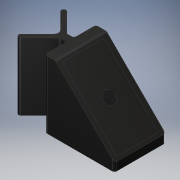
# Autodesk Inventor part: MainHousing
Saved by Autodesk Inventor 2019 (Build 230136000, 136)
## iProperties
Created: 2018-09-02
Part Number: MainHousing
Material: Generic
Document SubType Name: Modeling
Designer: Crater-Windows
Density: 1 g/cm^3
Appearance: Glossy - Black
Author: Crater-Windows
Autodesk Inventor part; units mm, degrees
ref_plane "YZ Plane" through (0, 0, 0) normal (1, 0, 0) x (0, 1, 0)
ref_plane "XZ Plane" through (0, 0, 0) normal (0, 1, 0) x (-1, 0, 0)
ref_plane "XY Plane" through (0, 0, 0) normal (0, 0, 1) x (1, 0, 0)
sketch "Sketch1" plane through (0, 0, 0) normal (1, 0, 0) x (0, 1, 0)
  line L0 (0, 0) -> (150, 0)
  line L1 (150, 0) -> (150, -110)
  line L2 (150, -110) -> (0, -110)
  line L3 (0, -110) -> (0, 0)
  dimension "d0" = 150
  dimension "d1" = 110
  constraints: 8 end point, 2 parallel, 1 horizontal, 1 perpendicular
  measures "d0" distance of L1.end L2.end
  measures "d1" distance of L0.end L1.end
extrude "Extrusion1" add sketch "Sketch1" along normal blind 150
sketch "Sketch2" plane through (0, 0, 0) normal (0, 0, 1) x (1, 0, 0)
  line L0 (0, 0) -> (0, 150) projected
  line L1 (0, 0) -> (150, 0) projected
  line L2 (150, 150) -> (150, 0) projected
  line L3 (0, 150) -> (150, 150) projected
  line L4 (0, 150) -> (150, 150) projected
  line L5 (22.7208, 150) -> (150, 22.7208)
  line L6 (22.7208, 150) -> (202.7208, 150) construction
  line L7 (150, 150) -> (150, 0) projected
  dimension "d4" = 45
  dimension "d6" = 180
  constraints: 4 end point, 2 point on line, 1 equal length, 1 horizontal
  measures "d4" angle of L5 L6
  measures "d6" distance of L5.start L5.end
extrude "Extrusion2" cut sketch "Sketch2" against normal blind 150 contours L3 L2 L5
shell "Shell1" thickness 6 removed faces 1 at (50, 0, -73.3333)
sketch "Sketch3" plane through (22.7208, 150, -110) normal (0.7071068, 0.7071068, 0) x (-0.7071068, 0.7071068, 0)
  line L0 (-7, 100) -> (-173, 100)
  line L1 (-173, 100) -> (-173, 10)
  line L2 (-173, 10) -> (-7, 10)
  line L3 (-7, 10) -> (-7, 100)
  line L4 (0, 110) -> (0, 0) projected
  line L5 (-180, 110) -> (0, 110) projected
  point P0 (-90, 110)
  dimension "d10" = 166
  dimension "d11" = 90
  dimension "d12" = 7
  dimension "d13" = 10
  constraints: 8 end point, 2 parallel, 1 horizontal, 1 perpendicular
  measures "d10" distance of L2.end L1.end
  measures "d11" distance of L1.end L0.end
  measures "d12" distance between parallel lines of L3 L4
  measures "d13" distance between parallel lines of L5 L0
extrude "Extrusion3" cut sketch "Sketch3" against normal blind 2.5
sketch "Sketch4" plane through (20.953, 148.2322, -110) normal (0.7071068, 0.7071068, 0) x (0, 0, 1)
  line L0 (0, 90) -> (110, 90) projected
  point P0 (55, 90)
  constraints: 1 midpoint
hole "Hole1" at (84.5926, 84.5926, -55) direction (-0.7071068, -0.7071068, 0) diameter 27 depth 12 tip angle 118
sketch "Sketch5" plane through (0, 150, 0) normal (0, 1, 0) x (1, 0, 0)
  line L0 (-64.0685, 97.4264) -> (-21.6421, 55)
  line L1 (-21.6421, 55) -> (-64.0685, 12.5736)
  line L2 (0, 0) -> (0, 110) projected
  line L3 (-64.0685, 97.4264) -> (-56.9975, 104.4975)
  line L4 (-56.9975, 104.4975) -> (-15, 62.5)
  line L5 (-15, 62.5) -> (0, 62.5)
  line L6 (-64.0685, 12.5736) -> (-56.9975, 5.5025)
  line L7 (-56.9975, 5.5025) -> (-15, 47.5)
  line L8 (-15, 47.5) -> (0, 47.5)
  line L9 (0, 110) -> (0, 0) projected
  arc A0 (-56.9975, 104.4975) -> (-64.0685, 97.4264) centre (-60.533, 100.9619) ccw
  arc A1 (-64.0685, 12.5736) -> (-56.9975, 5.5025) centre (-60.533, 9.0381) ccw
  dimension "d25" = 60
  dimension "d26" = 10
  dimension "d27" = 15
  dimension "d28" = 15
  dimension "d29" = 47.5
  constraints: 16 end point, 4 equal length, 4 parallel, 4 point on circle, 2 centre point, 2 perpendicular, 2 point on line, 2 tangent, 2 vertical alignment, 1 horizontal
  measures "d25" distance of L0.start L0.end
  measures "d26" distance between parallel lines of L4 L0
  measures "d27" distance of L4.end L5.end
  measures "d28" distance between parallel lines of L8 L5
  measures "d29" distance from line of L2.end L5
extrude "Extrusion4" add sketch "Sketch5" against normal blind 150
fillet "Fillet1" radius 10 1 edges at (-21.6421, 75, -55)
fillet "Fillet2" radius 5 10 edges at (0, 75, -47.5) (0, 75, -62.5) (-15, 75, -62.5) (-15, 75, -47.5) (0, 75, 0) (0, 75, -110) (150, 11.3604, -110) (150, 11.3604, 0) (20.2355, 144, -55) (22.7208, 150, -55)
chamfer "Chamfer1" distance 10 angle 45 4 edges at (144, 10.1177, -104) (144, 10.1177, -6) (6, 72, -6) (6, 72, -104)
fillet "Fillet3" radius 5 7 edges at (144, 20.2355, -55) (20.0778, 143.6194, -6) (17.0822, 144, -6) (77.85, 86.3855, -6) (20.0778, 143.6194, -104) (17.0822, 144, -104) (77.85, 86.3855, -104)
sketch "Sketch7" plane through (-35.7843, 0, -55) normal (0, -1, 0) x (1, 0, 0)
  arc A0 (185.7843, 50) -> (180.7843, 55) centre (180.7843, 50) ccw projected
  line L0 (40.7843, 55) -> (180.7843, 55) projected
  arc A1 (40.7843, 55) -> (35.7843, 50) centre (40.7843, 50) ccw projected
  line L1 (35.7843, 12.5) -> (35.7843, 50) projected
  arc A2 (30.7843, 7.5) -> (35.7843, 12.5) centre (30.7843, 12.5) ccw projected
  line L2 (30.7843, 7.5) -> (22.8553, 7.5) projected
  arc A3 (19.3198, 8.9645) -> (22.8553, 7.5) centre (22.8553, 12.5) ccw projected
  line L3 (19.3198, 8.9645) -> (-21.2132, 49.4975) projected
  arc A4 (-21.2132, 49.4975) -> (-28.2843, 42.4264) centre (-24.7487, 45.9619) ccw projected
  line L4 (-28.2843, 42.4264) -> (7.0711, 7.0711) projected
  arc A5 (7.0711, -7.0711) -> (7.0711, 7.0711) centre (0, 0) ccw projected
  line L5 (7.0711, -7.0711) -> (-28.2843, -42.4264) projected
  arc A6 (-28.2843, -42.4264) -> (-21.2132, -49.4975) centre (-24.7487, -45.9619) ccw projected
  line L6 (-21.2132, -49.4975) -> (19.3198, -8.9645) projected
  arc A7 (22.8553, -7.5) -> (19.3198, -8.9645) centre (22.8553, -12.5) ccw projected
  line L7 (22.8553, -7.5) -> (30.7843, -7.5) projected
  arc A8 (35.7843, -12.5) -> (30.7843, -7.5) centre (30.7843, -12.5) ccw projected
  line L8 (35.7843, -50) -> (35.7843, -12.5) projected
  arc A9 (35.7843, -50) -> (40.7843, -55) centre (40.7843, -50) ccw projected
  line L9 (40.7843, -55) -> (180.7843, -55) projected
  arc A10 (180.7843, -55) -> (185.7843, -50) centre (180.7843, -50) ccw projected
  line L10 (185.7843, 50) -> (185.7843, -50) projected
  line L11 (179.7843, 39) -> (179.7843, -39) projected
  line L12 (169.7843, -49) -> (179.7843, -39) projected
  line L13 (169.7843, -49) -> (51.7843, -49) projected
  line L14 (41.7843, -39) -> (51.7843, -49) projected
  line L15 (41.7843, -39) -> (41.7843, 39) projected
  line L16 (51.7843, 49) -> (41.7843, 39) projected
  line L17 (51.7843, 49) -> (169.7843, 49) projected
  line L18 (179.7843, 39) -> (169.7843, 49) projected
  point P0 (35.7843, 55)
  point P1 (41.7843, 49)
  point P2 (179.7843, 49)
  point P3 (179.7843, -49)
  point P4 (41.7843, -49)
  constraints: 4 horizontal alignment, 4 vertical alignment, 1 point on line
hole "Hole2" at (6, 0, -6) at (144, 0, -6) at (144, 0, -104) at (6, 0, -104) direction (0, 1, 0) diameter 5.3 depth 8.9
sketch "Sketch8" plane through (-12.9289, 150, -47.5) normal (0, 0, 1) x (1, 0, 0)
  line L0 (0, -150) -> (0, 0) projected
  line L1 (7.9289, -150) -> (0, -150) projected
  line L2 (7.9289, 0) -> (7.9289, -150) projected
  line L3 (0, 0) -> (7.9289, 0) projected
  line L4 (0, -30) -> (8, -30)
  line L5 (8, -30) -> (8, -50)
  line L6 (8, -50) -> (0, -50)
  line L7 (0, -50) -> (0, -30)
  line L8 (0, -100) -> (8, -100)
  line L9 (8, -100) -> (8, -120)
  line L10 (8, -120) -> (0, -120)
  line L11 (0, -120) -> (0, -100)
  point P0 (12.9289, -150)
  dimension "d45" = 8
  dimension "d46" = 20
  dimension "d47" = 8
  dimension "d48" = 20
  dimension "d49" = 30
  dimension "d50" = 30
  constraints: 16 end point, 4 parallel, 2 horizontal, 2 perpendicular, 2 vertical alignment
  measures "d45" distance of L5.end L6.end
  measures "d46" distance of L4.end L5.end
  measures "d47" distance of L9.end L10.end
  measures "d48" distance of L8.end L9.end
  measures "d49" distance between parallel lines of L4 L3
  measures "d50" distance between parallel lines of L1 L10
extrude "Extrusion5" cut sketch "Sketch8" against normal blind 150 contours L0 L8 L2 L10 | L2 L8 L9 L10 | L0 L4 L2 L6 | L2 L4 L5 L6
sketch "Sketch10" plane through (-35.7843, 0, -55) normal (0, -1, 0) x (1, 0, 0)
  circle A0 centre (179.7843, -49) radius 2.65 projected
  circle A1 centre (41.7843, 49) radius 2.65 projected
  circle A2 centre (179.7843, 49) radius 2.65 projected
  circle A3 centre (41.7843, -49) radius 2.65 projected
  arc A4 (185.7843, 50) -> (180.7843, 55) centre (180.7843, 50) ccw projected
  line L0 (40.7843, 55) -> (180.7843, 55) projected
  arc A5 (40.7843, 55) -> (35.7843, 50) centre (40.7843, 50) ccw projected
  line L1 (35.7843, 12.5) -> (35.7843, 50) projected
  arc A6 (30.7843, 7.5) -> (35.7843, 12.5) centre (30.7843, 12.5) ccw projected
  line L2 (30.7843, 7.5) -> (22.8553, 7.5) projected
  arc A7 (19.3198, 8.9645) -> (22.8553, 7.5) centre (22.8553, 12.5) ccw projected
  line L3 (19.3198, 8.9645) -> (-21.2132, 49.4975) projected
  arc A8 (-21.2132, 49.4975) -> (-28.2843, 42.4264) centre (-24.7487, 45.9619) ccw projected
  line L4 (-28.2843, 42.4264) -> (7.0711, 7.0711) projected
  arc A9 (7.0711, -7.0711) -> (7.0711, 7.0711) centre (0, 0) ccw projected
  line L5 (7.0711, -7.0711) -> (-28.2843, -42.4264) projected
  arc A10 (-28.2843, -42.4264) -> (-21.2132, -49.4975) centre (-24.7487, -45.9619) ccw projected
  line L6 (-21.2132, -49.4975) -> (19.3198, -8.9645) projected
  arc A11 (22.8553, -7.5) -> (19.3198, -8.9645) centre (22.8553, -12.5) ccw projected
  line L7 (22.8553, -7.5) -> (30.7843, -7.5) projected
  arc A12 (35.7843, -12.5) -> (30.7843, -7.5) centre (30.7843, -12.5) ccw projected
  line L8 (35.7843, -50) -> (35.7843, -12.5) projected
  arc A13 (35.7843, -50) -> (40.7843, -55) centre (40.7843, -50) ccw projected
  line L9 (40.7843, -55) -> (180.7843, -55) projected
  arc A14 (180.7843, -55) -> (185.7843, -50) centre (180.7843, -50) ccw projected
  line L10 (185.7843, 50) -> (185.7843, -50) projected
  line L11 (179.7843, 39) -> (179.7843, -39) projected
  line L12 (169.7843, -49) -> (179.7843, -39) projected
  line L13 (169.7843, -49) -> (51.7843, -49) projected
  line L14 (41.7843, -39) -> (51.7843, -49) projected
  line L15 (41.7843, -39) -> (41.7843, 39) projected
  line L16 (51.7843, 49) -> (41.7843, 39) projected
  line L17 (51.7843, 49) -> (169.7843, 49) projected
  line L18 (179.7843, 39) -> (169.7843, 49) projected
  point P0 (35.7843, 55)
extrude "Extrusion6" cut sketch "Sketch10" against normal blind 5
body "Solid1"
